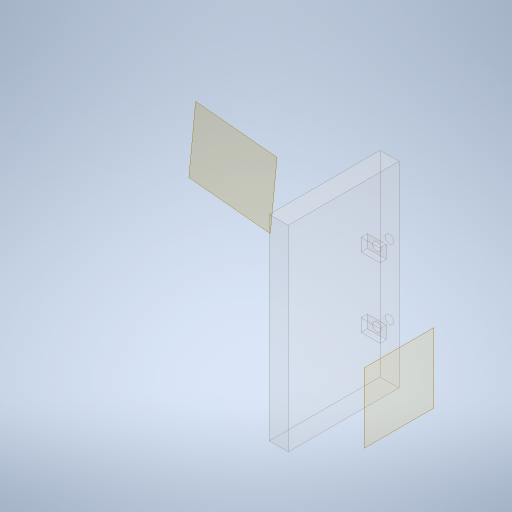
# Autodesk Inventor part: _head_adt_2
Saved by Autodesk Inventor 2024.3 (Build 283343000, 343)
## iProperties
Created: 2024-09-08
Part Number: _head_adt_2
Material: PMMA 플라스틱
Document SubType Name: Modeling
Designer: gretc
Density: 1.188 g/cm^3
Appearance: 폴리카보네이트 - 선명
Mass: 15.2748 g
Surface Area: 56.3349 cm^2
Volume: 12.8576 cm^3
Author: gretc
Autodesk Inventor part; units mm, degrees
ref_plane "YZ Plane" through (0, 0, 0) normal (1, 0, 0) x (0, 1, 0)
ref_plane "XZ Plane" through (0, 0, 0) normal (0, 1, 0) x (-1, 0, 0)
ref_plane "XY Plane" through (0, 0, 0) normal (0, 0, 1) x (1, 0, 0)
ref_plane "작업 평면2" through (-1.8693, 3.0801, 0) normal (0, 0, 1) x (0.9953009, -0.0968305, 0)
sketch "스케치1" plane through (-1.8693, 3.0801, 0) normal (0, 0, 1) x (0.9953009, -0.0968305, 0)
  line L0 (44.1285, 26.3164) -> (48.97, -23.4487) projected
  line L1 (49.551, -29.4205) -> (48.97, -23.4487) projected
  line L2 (55.5228, -28.8395) -> (-45.2017, -38.6387) projected
  line L3 (49.5193, 32.8692) -> (55.5228, -28.8395) projected
  line L4 (-51.2052, 23.0699) -> (49.5193, 32.8692) projected
  line L5 (44.1285, 26.3164) -> (43.5475, 32.2882) projected
  point P0 (2.1588, -2.8846)
extrude "돌출1" add sketch "스케치1" along normal blind 35
sketch "스케치2" plane through (-1.8693, 3.0801, 0) normal (0, 0, -1) x (-0.9953009, 0.0968305, 0)
  circle A0 centre (-48.7397, 9.9006) radius 1.35 projected
  circle A1 centre (-50.8699, -11.996) radius 1.35 projected
  point P0 (-2.1588, -2.8846)
extrude "돌출2" cut sketch "스케치2" against normal blind 5
ref_plane "작업 평면3" through (50.6, -31.0001, 0) normal (1, 0, 0) x (0, 0, -1)
sketch "스케치3" plane through (50.6, -31.0001, 0) normal (1, 0, 0) x (0, 0, -1)
  line L0 (-5, 40.5649) -> (-5, 37.8649) projected
  line L1 (-5, 18.5649) -> (-5, 15.8649) projected
  line L2 (-4, 0) -> (-4, 6) projected
  line L3 (-4, 1.65) -> (0, 1.65)
  line L4 (-4, 4.35) -> (0, 4.35)
  line L5 (-4, 37.2149) -> (-4, 41.2149)
  line L6 (-4, 41.2149) -> (-6, 41.2149)
  line L7 (-6, 41.2149) -> (-6, 37.2149)
  line L8 (-6, 37.2149) -> (-4, 37.2149)
  line L9 (-4, 37.2149) -> (-6, 41.2149) construction
  line L10 (-4, 41.2149) -> (-6, 37.2149) construction
  line L11 (-4, 15.2149) -> (-4, 19.2149)
  line L12 (-4, 19.2149) -> (-6, 19.2149)
  line L13 (-6, 19.2149) -> (-6, 15.2149)
  line L14 (-6, 15.2149) -> (-4, 15.2149)
  line L15 (-4, 15.2149) -> (-6, 19.2149) construction
  line L16 (-4, 19.2149) -> (-6, 15.2149) construction
  point P0 (0, 31.0001)
  point P1 (-5, 39.2149)
  point P2 (-5, 17.2149)
  dimension "d4" = 4
  dimension "d5" = 2
  dimension "d6" = 4
  constraints: 28 end point, 6 midpoint, 4 parallel, 3 perpendicular, 2 horizontal, 4 other
  measures "d4" distance of L5.start L5.end
  measures "d5" distance of L6.end L5.end
  measures "d6" distance of L11.start L11.end
extrude "돌출3" cut sketch "스케치3" against normal up to surface (6 mm away)
